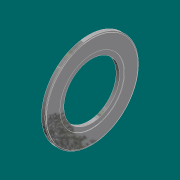
# Autodesk Inventor part: core_BA2542
Saved by Autodesk Inventor 2016 (Build 200138000, 138)
## iProperties
Category: PARTsolutions
Company: MISUMI
Created: 2016-05-01
Part Number: core_BA2542
Catalog Web Link: www.cadenas.de
Description: BA_ _ _ _core-Thrust Needle Roller Bearings with Retainers
Vendor: MISUMI
Document SubType Name: Modeling
Designer: psAdmin
Manufacturer: MISUMI
Mass: 20 g
Surface Area: 22.1482 cm^2
Volume: 1.67172 cm^3
Density: 11.9637 g/cm^3
Material: ステンレス鋼 440C
Appearance: 半つや出し
PSOL_IDENT_0: {$CADENAS_DATA\23d-libs\misumi\metric\12_bearing_holders\core_ba1024.prj},171 {VTYP=3D},{NB=core_BA2
PSOL_IDENT_1: 542},{LINA=core_BA2542},{NN=BA_ _ _ _core},{DATE=21.07.2015 12:46:34},{GEOMDATE=24.05.2010 00:00:00}
PSOL_IDENT_2: ,{VERSION=},{LINEID=60},{LINESUBID=-1},{WBVAR=}  {NB=core_BA2542},{LINA=core_BA2542},{KT=DUMMY},{TYP
PSOL_IDENT_3: E=BA2542},{MAT=SUJ2(52100 Bearing Steel)(1.3505_100Cr6) or Equivalent},{DD=25},{DDTOL=+0.250/+0.004}
PSOL_IDENT_4: ,{D=42},{DTOL=-0.130/-0.520},{B=2},{BTOL=0/-0.01},{F=41},{F1=29},{DD1=25},{DD1TOL=+0.370/+0.040},{D1=
PSOL_IDENT_5: 42},{D1TOL=-0.050/-0.440},{B1=1},{B1TOL=+0.05/-0.05},{MASS=21},{CA=14.7},{COA=58.0}
NN: BA_ _ _ _core
NT: Thrust Needle Roller Bearings with Retainers
NB: core_BA2542
NBSYN: core_$TYPE.
LINA: core_BA2542
TYPE: BA2542
MAT: SUJ2(52100 Bearing Steel)(1.3505_100Cr6) or Equivalent
DD: 25
DDTOL: +0.250/+0.004
D: 42
DTOL: -0.130/-0.520
B: 2
BTOL: 0/-0.01
F: 41
F1: 29
DD1: 25
DD1TOL: +0.370/+0.040
D1: 42
D1TOL: -0.050/-0.440
B1: 1
B1TOL: +0.05/-0.05
MASS: 21
CA: 14.7
COA: 58.0
SUPPLIER: MISUMI
ARTICLENO: core_BA2542
BOMINFO: core_BA2542
CREATOR: CADENAS GmbH
Title: core_BA2542
Author: Cadenas PARTsolutions
Comments: Thrust Needle Roller Bearings with Retainers
Autodesk Inventor part; units mm, degrees
sketch "Sketch_1" plane through (0, 0, 0) normal (0, 0, 1) x (1, 0, 0)
  line L0 (50, 0) -> (-50, 0)
  line L1 (-1, 20.5) -> (-1, 14.5)
  line L2 (-1, 14.5) -> (-0.75, 14.5)
  line L3 (-0.75, 14.5) -> (-0.75, 12.5)
  line L4 (-0.75, 12.5) -> (0.75, 12.5)
  line L5 (0.75, 12.5) -> (0.75, 14.5)
  line L6 (0.75, 14.5) -> (1, 14.5)
  line L7 (1, 14.5) -> (1, 20.5)
  line L8 (1, 20.5) -> (0.75, 20.5)
  line L9 (0.75, 20.5) -> (0.75, 21)
  line L10 (0.75, 21) -> (-0.75, 21)
  line L11 (-0.75, 21) -> (-0.75, 20.5)
  line L12 (-0.75, 20.5) -> (-1, 20.5)
  constraints: 26 end point
revolve "Revolution1" add sketch "Sketch_1" angle 360 about axis through (50, 0, 0) along (1, 0, 0)
ref_plane "core_to_washer_XY" through (0, 0, 0) normal (1, 0, 0) x (0, 0, -1)
ref_plane "core_to_washer_YZ" through (0, 0, 0) normal (0, 0, -1) x (0, 1, 0)
ref_plane "core_to_washer_ZX" through (0, 0, 0) normal (0, 1, 0) x (1, 0, 0)
ref_plane "core_to_washer1_XY" through (0, 0, 0) normal (-1, 0, 0) x (0, 0, -1)
ref_plane "core_to_washer1_YZ" through (0, 0, 0) normal (0, 0, -1) x (0, -1, 0)
ref_plane "core_to_washer1_ZX" through (0, 0, 0) normal (0, -1, 0) x (-1, 0, 0)
body "Solid1"
